Autodesk Fusion 360 part; units mm, degrees
(part 2 of 11)
  line L949 (170.706, 44.1166) -> (171.506, 44.1166)
  line L950 (171.506, 44.1166) -> (171.506, 43.1161)
  line L951 (171.506, 43.1161) -> (185.506, 43.1161)
  line L952 (185.506, 43.1161) -> (185.506, 44.1166)
  line L953 (185.506, 44.1166) -> (186.307, 44.1166)
  line L954 (186.307, 44.1166) -> (186.307, 47.2172)
  line L955 (186.307, 47.2172) -> (185.506, 47.2172)
  line L956 (185.506, 47.2172) -> (185.506, 53.0172)
  line L957 (185.506, 53.0172) -> (186.307, 53.0172)
  line L958 (186.307, 53.0172) -> (186.307, 56.1164)
  line L959 (186.307, 56.1164) -> (185.506, 56.1164)
  line L960 (185.506, 56.1164) -> (185.506, 57.1168)
  line L961 (185.506, 57.1168) -> (171.506, 57.1168)
  line L962 (190.556, 57.1168) -> (190.556, 56.1164)
  line L963 (190.556, 56.1164) -> (189.756, 56.1164)
  line L964 (189.756, 56.1164) -> (189.756, 53.0172)
  line L965 (189.756, 53.0172) -> (190.556, 53.0172)
  line L966 (190.556, 53.0172) -> (190.556, 47.2172)
  line L967 (190.556, 47.2172) -> (189.756, 47.2172)
  line L968 (189.756, 47.2172) -> (189.756, 44.1166)
  line L969 (189.756, 44.1166) -> (190.556, 44.1166)
  line L970 (190.556, 44.1166) -> (190.556, 43.1161)
  line L971 (190.556, 43.1161) -> (204.556, 43.1161)
  line L972 (204.556, 43.1161) -> (204.556, 44.1166)
  line L973 (204.556, 44.1166) -> (205.357, 44.1166)
  line L974 (205.357, 44.1166) -> (205.357, 47.2172)
  line L975 (205.357, 47.2172) -> (204.556, 47.2172)
  line L976 (204.556, 47.2172) -> (204.556, 53.0172)
  line L977 (204.556, 53.0172) -> (205.357, 53.0172)
  line L978 (205.357, 53.0172) -> (205.357, 56.1164)
  line L979 (205.357, 56.1164) -> (204.556, 56.1164)
  line L980 (204.556, 56.1164) -> (204.556, 57.1168)
  line L981 (204.556, 57.1168) -> (190.556, 57.1168)
  line L982 (209.606, 57.1168) -> (209.606, 56.1164)
  line L983 (209.606, 56.1164) -> (208.806, 56.1164)
  line L984 (208.806, 56.1164) -> (208.806, 53.0172)
  line L985 (208.806, 53.0172) -> (209.606, 53.0172)
  line L986 (209.606, 53.0172) -> (209.606, 47.2172)
  line L987 (209.606, 47.2172) -> (208.806, 47.2172)
  line L988 (208.806, 47.2172) -> (208.806, 44.1166)
  line L989 (208.806, 44.1166) -> (209.606, 44.1166)
  line L990 (209.606, 44.1166) -> (209.606, 43.1161)
  line L991 (209.606, 43.1161) -> (223.606, 43.1161)
  line L992 (223.606, 43.1161) -> (223.606, 44.1166)
  line L993 (223.606, 44.1166) -> (224.407, 44.1166)
  line L994 (224.407, 44.1166) -> (224.407, 47.2172)
  line L995 (224.407, 47.2172) -> (223.606, 47.2172)
  line L996 (223.606, 47.2172) -> (223.606, 53.0172)
  line L997 (223.606, 53.0172) -> (224.407, 53.0172)
  line L998 (224.407, 53.0172) -> (224.407, 56.1164)
  line L999 (224.407, 56.1164) -> (223.606, 56.1164)
  line L1000 (223.606, 56.1164) -> (223.606, 57.1168)
  line L1001 (223.606, 57.1168) -> (209.606, 57.1168)
  line L1002 (228.656, 57.1168) -> (228.656, 56.1164)
  line L1003 (228.656, 56.1164) -> (227.856, 56.1164)
  line L1004 (227.856, 56.1164) -> (227.856, 53.0172)
  line L1005 (227.856, 53.0172) -> (228.656, 53.0172)
  line L1006 (228.656, 53.0172) -> (228.656, 47.2172)
  line L1007 (228.656, 47.2172) -> (227.856, 47.2172)
  line L1008 (227.856, 47.2172) -> (227.856, 44.1166)
  line L1009 (227.856, 44.1166) -> (228.656, 44.1166)
  line L1010 (228.656, 44.1166) -> (228.656, 43.1161)
  line L1011 (228.656, 43.1161) -> (242.656, 43.1161)
  line L1012 (242.656, 43.1161) -> (242.656, 44.1166)
  line L1013 (242.656, 44.1166) -> (243.457, 44.1166)
  line L1014 (243.457, 44.1166) -> (243.457, 47.2172)
  line L1015 (243.457, 47.2172) -> (242.656, 47.2172)
  line L1016 (242.656, 47.2172) -> (242.656, 53.0172)
  line L1017 (242.656, 53.0172) -> (243.457, 53.0172)
  line L1018 (243.457, 53.0172) -> (243.457, 56.1164)
  line L1019 (243.457, 56.1164) -> (242.656, 56.1164)
  line L1020 (242.656, 56.1164) -> (242.656, 57.1168)
  line L1021 (242.656, 57.1168) -> (228.656, 57.1168)
  line L1022 (247.706, 57.1168) -> (247.706, 56.1164)
  line L1023 (247.706, 56.1164) -> (246.906, 56.1164)
  line L1024 (246.906, 56.1164) -> (246.906, 53.0172)
  line L1025 (246.906, 53.0172) -> (247.706, 53.0172)
  line L1026 (247.706, 53.0172) -> (247.706, 47.2172)
  line L1027 (247.706, 47.2172) -> (246.906, 47.2172)
  line L1028 (246.906, 47.2172) -> (246.906, 44.1166)
  line L1029 (246.906, 44.1166) -> (247.706, 44.1166)
  line L1030 (247.706, 44.1166) -> (247.706, 43.1161)
  line L1031 (247.706, 43.1161) -> (261.706, 43.1161)
  line L1032 (261.706, 43.1161) -> (261.706, 44.1166)
  line L1033 (261.706, 44.1166) -> (262.507, 44.1166)
  line L1034 (262.507, 44.1166) -> (262.507, 47.2172)
  line L1035 (262.507, 47.2172) -> (261.706, 47.2172)
  line L1036 (261.706, 47.2172) -> (261.706, 53.0172)
  line L1037 (261.706, 53.0172) -> (262.507, 53.0172)
  line L1038 (262.507, 53.0172) -> (262.507, 56.1164)
  line L1039 (262.507, 56.1164) -> (261.706, 56.1164)
  line L1040 (261.706, 56.1164) -> (261.706, 57.1168)
  line L1041 (261.706, 57.1168) -> (247.706, 57.1168)
  line L1042 (357.244, 57.1168) -> (357.244, 56.1164)
  line L1043 (357.244, 56.1164) -> (356.443, 56.1164)
  line L1044 (356.443, 56.1164) -> (356.443, 53.0172)
  line L1045 (356.443, 53.0172) -> (357.244, 53.0172)
  line L1046 (357.244, 53.0172) -> (357.244, 47.2172)
  line L1047 (357.244, 47.2172) -> (356.443, 47.2172)
  line L1048 (356.443, 47.2172) -> (356.443, 44.1166)
  line L1049 (356.443, 44.1166) -> (357.244, 44.1166)
  line L1050 (357.244, 44.1166) -> (357.244, 43.1161)
  line L1051 (357.244, 43.1161) -> (371.246, 43.1161)
  line L1052 (371.246, 43.1161) -> (371.246, 44.1166)
  line L1053 (371.246, 44.1166) -> (372.043, 44.1166)
  line L1054 (372.043, 44.1166) -> (372.043, 47.2172)
  line L1055 (372.043, 47.2172) -> (371.246, 47.2172)
  line L1056 (371.246, 47.2172) -> (371.246, 53.0172)
  line L1057 (371.246, 53.0172) -> (372.043, 53.0172)
  line L1058 (372.043, 53.0172) -> (372.043, 56.1164)
  line L1059 (372.043, 56.1164) -> (371.246, 56.1164)
  line L1060 (371.246, 56.1164) -> (371.246, 57.1168)
  line L1061 (371.246, 57.1168) -> (357.244, 57.1168)
  line L1062 (376.294, 57.1168) -> (376.294, 56.1164)
  line L1063 (376.294, 56.1164) -> (375.493, 56.1164)
  line L1064 (375.493, 56.1164) -> (375.493, 53.0172)
  line L1065 (375.493, 53.0172) -> (376.294, 53.0172)
  line L1066 (376.294, 53.0172) -> (376.294, 47.2172)
  line L1067 (376.294, 47.2172) -> (375.493, 47.2172)
  line L1068 (375.493, 47.2172) -> (375.493, 44.1166)
  line L1069 (375.493, 44.1166) -> (376.294, 44.1166)
  line L1070 (376.294, 44.1166) -> (376.294, 43.1161)
  line L1071 (376.294, 43.1161) -> (390.296, 43.1161)
  line L1072 (390.296, 43.1161) -> (390.296, 44.1166)
  line L1073 (390.296, 44.1166) -> (391.093, 44.1166)
  line L1074 (391.093, 44.1166) -> (391.093, 47.2172)
  line L1075 (391.093, 47.2172) -> (390.296, 47.2172)
  line L1076 (390.296, 47.2172) -> (390.296, 53.0172)
  line L1077 (390.296, 53.0172) -> (391.093, 53.0172)
  line L1078 (391.093, 53.0172) -> (391.093, 56.1164)
  line L1079 (391.093, 56.1164) -> (390.296, 56.1164)
  line L1080 (390.296, 56.1164) -> (390.296, 57.1168)
  line L1081 (390.296, 57.1168) -> (376.294, 57.1168)
  line L1082 (395.344, 57.1168) -> (395.344, 56.1164)
  line L1083 (395.344, 56.1164) -> (394.543, 56.1164)
  line L1084 (394.543, 56.1164) -> (394.543, 53.0172)
  line L1085 (394.543, 53.0172) -> (395.344, 53.0172)
  line L1086 (395.344, 53.0172) -> (395.344, 47.2172)
  line L1087 (395.344, 47.2172) -> (394.543, 47.2172)
  line L1088 (394.543, 47.2172) -> (394.543, 44.1166)
  line L1089 (394.543, 44.1166) -> (395.344, 44.1166)
  line L1090 (395.344, 44.1166) -> (395.344, 43.1161)
  line L1091 (395.344, 43.1161) -> (409.346, 43.1161)
  line L1092 (409.346, 43.1161) -> (409.346, 44.1166)
  line L1093 (409.346, 44.1166) -> (410.143, 44.1166)
  line L1094 (410.143, 44.1166) -> (410.143, 47.2172)
  line L1095 (410.143, 47.2172) -> (409.346, 47.2172)
  line L1096 (409.346, 47.2172) -> (409.346, 53.0172)
  line L1097 (409.346, 53.0172) -> (410.143, 53.0172)
  line L1098 (410.143, 53.0172) -> (410.143, 56.1164)
  line L1099 (410.143, 56.1164) -> (409.346, 56.1164)
  line L1100 (409.346, 56.1164) -> (409.346, 57.1168)
  line L1101 (409.346, 57.1168) -> (395.344, 57.1168)
  line L1102 (275.638, 75.741) -> (275.638, 74.9169)
  line L1103 (275.638, 74.9169) -> (269.368, 74.9169)
  line L1104 (269.368, 74.9169) -> (269.368, 73.1919)
  line L1105 (269.368, 73.1919) -> (268.388, 73.1919)
  line L1106 (268.388, 73.1919) -> (268.388, 69.8913)
  line L1107 (268.388, 69.8913) -> (269.368, 69.8913)
  line L1108 (269.368, 69.8913) -> (269.368, 68.1662)
  line L1109 (269.368, 68.1662) -> (273.837, 68.1662)
  line L1110 (273.837, 68.1662) -> (273.837, 66.6418)
  line L1111 (273.837, 66.6418) -> (273.237, 66.6418)
  line L1112 (273.237, 66.6418) -> (273.237, 67.4412)
  line L1113 (273.237, 67.4412) -> (270.137, 67.4412)
  line L1114 (270.137, 67.4412) -> (270.137, 66.6418)
  line L1115 (270.137, 66.6418) -> (269.138, 66.6418)
  line L1116 (269.138, 66.6418) -> (269.138, 52.6411)
  line L1117 (269.138, 52.6411) -> (270.137, 52.6411)
  line L1118 (270.137, 52.6411) -> (270.137, 51.8418)
  line L1119 (270.137, 51.8418) -> (273.237, 51.8418)
  line L1120 (273.237, 51.8418) -> (273.237, 52.6411)
  line L1121 (273.237, 52.6411) -> (273.837, 52.6411)
  line L1122 (273.837, 52.6411) -> (273.837, 51.1168)
  line L1123 (273.837, 51.1168) -> (269.368, 51.1168)
  line L1124 (269.368, 51.1168) -> (269.368, 49.3917)
  line L1125 (269.368, 49.3917) -> (268.388, 49.3917)
  line L1126 (268.388, 49.3917) -> (268.388, 46.0911)
  line L1127 (268.388, 46.0911) -> (269.368, 46.0911)
  line L1128 (269.368, 46.0911) -> (269.368, 44.366)
  line L1129 (269.368, 44.366) -> (275.638, 44.366)
  line L1130 (275.638, 44.366) -> (275.638, 43.542)
  line L1131 (275.638, 43.542) -> (278.438, 43.542)
  line L1132 (278.438, 43.542) -> (278.438, 44.366)
  line L1133 (278.438, 44.366) -> (281.667, 44.366)
  line L1134 (281.667, 44.366) -> (281.667, 46.0911)
  line L1135 (281.667, 46.0911) -> (282.587, 46.0911)
  line L1136 (282.587, 46.0911) -> (282.587, 49.3917)
  line L1137 (282.587, 49.3917) -> (281.667, 49.3917)
  line L1138 (281.667, 49.3917) -> (281.667, 51.1168)
  line L1139 (281.667, 51.1168) -> (278.438, 51.1168)
  line L1140 (278.438, 51.1168) -> (278.438, 52.6411)
  line L1141 (278.438, 52.6411) -> (279.038, 52.6411)
  line L1142 (279.038, 52.6411) -> (279.038, 51.8418)
  line L1143 (279.038, 51.8418) -> (282.138, 51.8418)
  line L1144 (282.138, 51.8418) -> (282.138, 52.6411)
  line L1145 (282.138, 52.6411) -> (283.137, 52.6411)
  line L1146 (283.137, 52.6411) -> (283.137, 66.6418)
  line L1147 (283.137, 66.6418) -> (282.138, 66.6418)
  line L1148 (282.138, 66.6418) -> (282.138, 67.4412)
  line L1149 (282.138, 67.4412) -> (279.038, 67.4412)
  line L1150 (279.038, 67.4412) -> (279.038, 66.6418)
  line L1151 (279.038, 66.6418) -> (278.438, 66.6418)
  line L1152 (278.438, 66.6418) -> (278.438, 68.1662)
  line L1153 (278.438, 68.1662) -> (281.667, 68.1662)
  line L1154 (281.667, 68.1662) -> (281.667, 69.8913)
  line L1155 (281.667, 69.8913) -> (282.587, 69.8913)
  line L1156 (282.587, 69.8913) -> (282.587, 73.1919)
  line L1157 (282.587, 73.1919) -> (281.667, 73.1919)
  line L1158 (281.667, 73.1919) -> (281.667, 74.9169)
  line L1159 (281.667, 74.9169) -> (278.438, 74.9169)
  line L1160 (278.438, 74.9169) -> (278.438, 75.741)
  line L1161 (278.438, 75.741) -> (275.638, 75.741)
  line L1162 (420.896, 75.741) -> (420.896, 74.9169)
  line L1163 (420.896, 74.9169) -> (414.623, 74.9169)
  line L1164 (414.623, 74.9169) -> (414.623, 73.1919)
  line L1165 (414.623, 73.1919) -> (413.646, 73.1919)
  line L1166 (413.646, 73.1919) -> (413.646, 69.8913)
  line L1167 (413.646, 69.8913) -> (414.623, 69.8913)
  line L1168 (414.623, 69.8913) -> (414.623, 68.1662)
  line L1169 (414.623, 68.1662) -> (419.093, 68.1662)
  line L1170 (419.093, 68.1662) -> (419.093, 66.6418)
  line L1171 (419.093, 66.6418) -> (418.497, 66.6418)
  line L1172 (418.497, 66.6418) -> (418.497, 67.4412)
  line L1173 (418.497, 67.4412) -> (415.396, 67.4412)
  line L1174 (415.396, 67.4412) -> (415.396, 66.6418)
  line L1175 (415.396, 66.6418) -> (414.394, 66.6418)
  line L1176 (414.394, 66.6418) -> (414.394, 52.6411)
  line L1177 (414.394, 52.6411) -> (415.396, 52.6411)
  line L1178 (415.396, 52.6411) -> (415.396, 51.8418)
  line L1179 (415.396, 51.8418) -> (418.497, 51.8418)
  line L1180 (418.497, 51.8418) -> (418.497, 52.6411)
  line L1181 (418.497, 52.6411) -> (419.093, 52.6411)
  line L1182 (419.093, 52.6411) -> (419.093, 51.1168)
  line L1183 (419.093, 51.1168) -> (414.623, 51.1168)
  line L1184 (414.623, 51.1168) -> (414.623, 49.3917)
  line L1185 (414.623, 49.3917) -> (413.646, 49.3917)
  line L1186 (413.646, 49.3917) -> (413.646, 46.0911)
  line L1187 (413.646, 46.0911) -> (414.623, 46.0911)
  line L1188 (414.623, 46.0911) -> (414.623, 44.366)
  line L1189 (414.623, 44.366) -> (420.896, 44.366)
  line L1190 (420.896, 44.366) -> (420.896, 43.542)
  line L1191 (420.896, 43.542) -> (423.693, 43.542)
  line L1192 (423.693, 43.542) -> (423.693, 44.366)
  line L1193 (423.693, 44.366) -> (426.925, 44.366)
  line L1194 (426.925, 44.366) -> (426.925, 46.0911)
  line L1195 (426.925, 46.0911) -> (427.845, 46.0911)
  line L1196 (427.845, 46.0911) -> (427.845, 49.3917)
  line L1197 (427.845, 49.3917) -> (426.925, 49.3917)
  line L1198 (426.925, 49.3917) -> (426.925, 51.1168)
  line L1199 (426.925, 51.1168) -> (423.693, 51.1168)
  line L1200 (423.693, 51.1168) -> (423.693, 52.6411)
  line L1201 (423.693, 52.6411) -> (424.293, 52.6411)
  line L1202 (424.293, 52.6411) -> (424.293, 51.8418)
  line L1203 (424.293, 51.8418) -> (427.394, 51.8418)
  line L1204 (427.394, 51.8418) -> (427.394, 52.6411)
  line L1205 (427.394, 52.6411) -> (428.396, 52.6411)
  line L1206 (428.396, 52.6411) -> (428.396, 66.6418)
  line L1207 (428.396, 66.6418) -> (427.394, 66.6418)
  line L1208 (427.394, 66.6418) -> (427.394, 67.4412)
  line L1209 (427.394, 67.4412) -> (424.293, 67.4412)
  line L1210 (424.293, 67.4412) -> (424.293, 66.6418)
  line L1211 (424.293, 66.6418) -> (423.693, 66.6418)
  line L1212 (423.693, 66.6418) -> (423.693, 68.1662)
  line L1213 (423.693, 68.1662) -> (426.925, 68.1662)
  line L1214 (426.925, 68.1662) -> (426.925, 69.8913)
  line L1215 (426.925, 69.8913) -> (427.845, 69.8913)
  line L1216 (427.845, 69.8913) -> (427.845, 73.1919)
  line L1217 (427.845, 73.1919) -> (426.925, 73.1919)
  line L1218 (426.925, 73.1919) -> (426.925, 74.9169)
  line L1219 (426.925, 74.9169) -> (423.693, 74.9169)
  line L1220 (423.693, 74.9169) -> (423.693, 75.741)
  line L1221 (423.693, 75.741) -> (420.896, 75.741)
  line L1222 (9.5815, 76.1668) -> (9.5815, 75.1664)
  line L1223 (9.5815, 75.1664) -> (8.7808, 75.1664)
  line L1224 (8.7809, 75.1664) -> (8.7809, 72.0672)
  line L1225 (8.7809, 72.0672) -> (9.5815, 72.0672)
  line L1226 (9.5815, 72.0672) -> (9.5815, 66.2672)
  line L1227 (9.5815, 66.2672) -> (8.7808, 66.2672)
  line L1228 (8.7809, 66.2672) -> (8.7809, 63.1666)
  line L1229 (8.7809, 63.1666) -> (9.5815, 63.1666)
  line L1230 (9.5815, 63.1666) -> (9.5815, 62.1661)
  line L1231 (9.5815, 62.1661) -> (23.581, 62.1661)
  line L1232 (23.581, 62.1661) -> (23.581, 63.1666)
  line L1233 (23.581, 63.1666) -> (24.3816, 63.1666)
  line L1234 (24.3816, 63.1666) -> (24.3816, 66.2672)
  line L1235 (24.3816, 66.2672) -> (23.581, 66.2672)
  line L1236 (23.581, 66.2672) -> (23.581, 72.0672)
  line L1237 (23.581, 72.0672) -> (24.3816, 72.0672)
  line L1238 (24.3816, 72.0672) -> (24.3816, 75.1664)
  line L1239 (24.3816, 75.1664) -> (23.581, 75.1664)
  line L1240 (23.581, 75.1664) -> (23.581, 76.1668)
  line L1241 (23.581, 76.1668) -> (9.5815, 76.1668)
  line L1242 (33.394, 76.1668) -> (33.394, 75.1664)
  line L1243 (33.394, 75.1664) -> (32.5947, 75.1664)
  line L1244 (32.5947, 75.1664) -> (32.5947, 72.0672)
  line L1245 (32.5947, 72.0672) -> (33.394, 72.0672)
  line L1246 (33.394, 72.0672) -> (33.394, 66.2672)
  line L1247 (33.394, 66.2672) -> (32.5947, 66.2672)
  line L1248 (32.5947, 66.2672) -> (32.5947, 63.1666)
  line L1249 (32.5947, 63.1666) -> (33.394, 63.1666)
  line L1250 (33.394, 63.1666) -> (33.394, 62.1661)
  line L1251 (33.394, 62.1661) -> (47.395, 62.1661)
  line L1252 (47.395, 62.1661) -> (47.395, 63.1666)
  line L1253 (47.395, 63.1666) -> (48.194, 63.1666)
  line L1254 (48.194, 63.1666) -> (48.194, 66.2672)
  line L1255 (48.194, 66.2672) -> (47.395, 66.2672)
  line L1256 (47.395, 66.2672) -> (47.395, 72.0672)
  line L1257 (47.395, 72.0672) -> (48.194, 72.0672)
  line L1258 (48.194, 72.0672) -> (48.194, 75.1664)
  line L1259 (48.194, 75.1664) -> (47.395, 75.1664)
  line L1260 (47.395, 75.1664) -> (47.395, 76.1668)
  line L1261 (47.395, 76.1668) -> (33.394, 76.1668)
  line L1262 (52.4439, 76.1668) -> (52.4439, 75.1664)
  line L1263 (52.4439, 75.1664) -> (51.6449, 75.1664)
  line L1264 (51.6449, 75.1664) -> (51.6449, 72.0672)
  line L1265 (51.6449, 72.0672) -> (52.4439, 72.0672)
  line L1266 (52.4439, 72.0672) -> (52.4439, 66.2672)
  line L1267 (52.4439, 66.2672) -> (51.6449, 66.2672)
  line L1268 (51.6449, 66.2672) -> (51.6449, 63.1666)
  line L1269 (51.6449, 63.1666) -> (52.4439, 63.1666)
  line L1270 (52.4439, 63.1666) -> (52.4439, 62.1661)
  line L1271 (52.4439, 62.1661) -> (66.445, 62.1661)
  line L1272 (66.445, 62.1661) -> (66.445, 63.1666)
  line L1273 (66.445, 63.1666) -> (67.244, 63.1666)
  line L1274 (67.244, 63.1666) -> (67.244, 66.2672)
  line L1275 (67.244, 66.2672) -> (66.445, 66.2672)
  line L1276 (66.445, 66.2672) -> (66.445, 72.0672)
  line L1277 (66.445, 72.0672) -> (67.244, 72.0672)
  line L1278 (67.244, 72.0672) -> (67.244, 75.1664)
  line L1279 (67.244, 75.1664) -> (66.445, 75.1664)
  line L1280 (66.445, 75.1664) -> (66.445, 76.1668)
  line L1281 (66.445, 76.1668) -> (52.4439, 76.1668)
  line L1282 (71.4939, 76.1668) -> (71.4939, 75.1664)
  line L1283 (71.4939, 75.1664) -> (70.6949, 75.1664)
  line L1284 (70.6949, 75.1664) -> (70.6949, 72.0672)
  line L1285 (70.6949, 72.0672) -> (71.4939, 72.0672)
  line L1286 (71.4939, 72.0672) -> (71.4939, 66.2672)
  line L1287 (71.4939, 66.2672) -> (70.6949, 66.2672)
  line L1288 (70.6949, 66.2672) -> (70.6949, 63.1666)
  line L1289 (70.6949, 63.1666) -> (71.4939, 63.1666)
  line L1290 (71.4939, 63.1666) -> (71.4939, 62.1661)
  line L1291 (71.4939, 62.1661) -> (85.4936, 62.1661)
  line L1292 (85.4936, 62.1661) -> (85.4936, 63.1666)
  line L1293 (85.4936, 63.1666) -> (86.294, 63.1666)
  line L1294 (86.294, 63.1666) -> (86.294, 66.2672)
  line L1295 (86.294, 66.2672) -> (85.4936, 66.2672)
  line L1296 (85.4936, 66.2672) -> (85.4936, 72.0672)
  line L1297 (85.4936, 72.0672) -> (86.294, 72.0672)
  line L1298 (86.294, 72.0672) -> (86.294, 75.1664)
  line L1299 (86.294, 75.1664) -> (85.4936, 75.1664)
  line L1300 (85.4936, 75.1664) -> (85.4936, 76.1668)
  line L1301 (85.4936, 76.1668) -> (71.4939, 76.1668)
  line L1302 (90.5439, 76.1668) -> (90.5439, 75.1664)
  line L1303 (90.5439, 75.1664) -> (89.7435, 75.1664)
  line L1304 (89.7435, 75.1664) -> (89.7435, 72.0672)
  line L1305 (89.7435, 72.0672) -> (90.5439, 72.0672)
  line L1306 (90.5439, 72.0672) -> (90.5439, 66.2672)
  line L1307 (90.5439, 66.2672) -> (89.7435, 66.2672)
  line L1308 (89.7435, 66.2672) -> (89.7435, 63.1666)
  line L1309 (89.7435, 63.1666) -> (90.5439, 63.1666)
  line L1310 (90.5439, 63.1666) -> (90.5439, 62.1661)
  line L1311 (90.5439, 62.1661) -> (104.544, 62.1661)
  line L1312 (104.544, 62.1661) -> (104.544, 63.1666)
  line L1313 (104.544, 63.1666) -> (105.344, 63.1666)
  line L1314 (105.344, 63.1666) -> (105.344, 66.2672)
  line L1315 (105.344, 66.2672) -> (104.544, 66.2672)
  line L1316 (104.544, 66.2672) -> (104.544, 72.0672)
  line L1317 (104.544, 72.0672) -> (105.344, 72.0672)
  line L1318 (105.344, 72.0672) -> (105.344, 75.1664)
  line L1319 (105.344, 75.1664) -> (104.544, 75.1664)
  line L1320 (104.544, 75.1664) -> (104.544, 76.1668)
  line L1321 (104.544, 76.1668) -> (90.5439, 76.1668)
  line L1322 (109.594, 76.1668) -> (109.594, 75.1664)
  line L1323 (109.594, 75.1664) -> (108.793, 75.1664)
  line L1324 (108.793, 75.1664) -> (108.793, 72.0672)
  line L1325 (108.793, 72.0672) -> (109.594, 72.0672)
  line L1326 (109.594, 72.0672) -> (109.594, 66.2672)
  line L1327 (109.594, 66.2672) -> (108.793, 66.2672)
  line L1328 (108.793, 66.2672) -> (108.793, 63.1666)
  line L1329 (108.793, 63.1666) -> (109.594, 63.1666)
  line L1330 (109.594, 63.1666) -> (109.594, 62.1661)
  line L1331 (109.594, 62.1661) -> (123.595, 62.1661)
  line L1332 (123.595, 62.1661) -> (123.595, 63.1666)
  line L1333 (123.595, 63.1666) -> (124.394, 63.1666)
  line L1334 (124.394, 63.1666) -> (124.394, 66.2672)
  line L1335 (124.394, 66.2672) -> (123.595, 66.2672)
  line L1336 (123.595, 66.2672) -> (123.595, 72.0672)
  line L1337 (123.595, 72.0672) -> (124.394, 72.0672)
  line L1338 (124.394, 72.0672) -> (124.394, 75.1664)
  line L1339 (124.394, 75.1664) -> (123.595, 75.1664)
  line L1340 (123.595, 75.1664) -> (123.595, 76.1668)
  line L1341 (123.595, 76.1668) -> (109.594, 76.1668)
  line L1342 (128.644, 76.1668) -> (128.644, 75.1664)
  line L1343 (128.644, 75.1664) -> (127.843, 75.1664)
  line L1344 (127.843, 75.1664) -> (127.843, 72.0672)
  line L1345 (127.843, 72.0672) -> (128.644, 72.0672)
  line L1346 (128.644, 72.0672) -> (128.644, 66.2672)
  line L1347 (128.644, 66.2672) -> (127.843, 66.2672)
  line L1348 (127.843, 66.2672) -> (127.843, 63.1666)
  line L1349 (127.843, 63.1666) -> (128.644, 63.1666)
  line L1350 (128.644, 63.1666) -> (128.644, 62.1661)
  line L1351 (128.644, 62.1661) -> (142.644, 62.1661)
  line L1352 (142.644, 62.1661) -> (142.644, 63.1666)
  line L1353 (142.644, 63.1666) -> (143.444, 63.1666)
  line L1354 (143.444, 63.1666) -> (143.444, 66.2672)
  line L1355 (143.444, 66.2672) -> (142.644, 66.2672)
  line L1356 (142.644, 66.2672) -> (142.644, 72.0672)
  line L1357 (142.644, 72.0672) -> (143.444, 72.0672)
  line L1358 (143.444, 72.0672) -> (143.444, 75.1664)
  line L1359 (143.444, 75.1664) -> (142.644, 75.1664)
  line L1360 (142.644, 75.1664) -> (142.644, 76.1668)
  line L1361 (142.644, 76.1668) -> (128.644, 76.1668)
  line L1362 (147.694, 76.1668) -> (147.694, 75.1664)
  line L1363 (147.694, 75.1664) -> (146.893, 75.1664)
  line L1364 (146.893, 75.1664) -> (146.893, 72.0672)
  line L1365 (146.893, 72.0672) -> (147.694, 72.0672)
  line L1366 (147.694, 72.0672) -> (147.694, 66.2672)
  line L1367 (147.694, 66.2672) -> (146.893, 66.2672)
  line L1368 (146.893, 66.2672) -> (146.893, 63.1666)
  line L1369 (146.893, 63.1666) -> (147.694, 63.1666)
  line L1370 (147.694, 63.1666) -> (147.694, 62.1661)
  line L1371 (147.694, 62.1661) -> (161.695, 62.1661)
  line L1372 (161.695, 62.1661) -> (161.695, 63.1666)
  line L1373 (161.695, 63.1666) -> (162.494, 63.1666)
  line L1374 (162.494, 63.1666) -> (162.494, 66.2672)
  line L1375 (162.494, 66.2672) -> (161.695, 66.2672)
  line L1376 (161.695, 66.2672) -> (161.695, 72.0672)
  line L1377 (161.695, 72.0672) -> (162.494, 72.0672)
  line L1378 (162.494, 72.0672) -> (162.494, 75.1664)
  line L1379 (162.494, 75.1664) -> (161.695, 75.1664)
  line L1380 (161.695, 75.1664) -> (161.695, 76.1668)
  line L1381 (161.695, 76.1668) -> (147.694, 76.1668)
  line L1382 (166.744, 76.1668) -> (166.744, 75.1664)
  line L1383 (166.744, 75.1664) -> (165.945, 75.1664)
  line L1384 (165.945, 75.1664) -> (165.945, 72.0672)
  line L1385 (165.945, 72.0672) -> (166.744, 72.0672)
  line L1386 (166.744, 72.0672) -> (166.744, 66.2672)
  line L1387 (166.744, 66.2672) -> (165.945, 66.2672)
  line L1388 (165.945, 66.2672) -> (165.945, 63.1666)
  line L1389 (165.945, 63.1666) -> (166.744, 63.1666)
  line L1390 (166.744, 63.1666) -> (166.744, 62.1661)
  line L1391 (166.744, 62.1661) -> (180.745, 62.1661)
  line L1392 (180.745, 62.1661) -> (180.745, 63.1666)
  line L1393 (180.745, 63.1666) -> (181.544, 63.1666)
  line L1394 (181.544, 63.1666) -> (181.544, 66.2672)
  line L1395 (181.544, 66.2672) -> (180.745, 66.2672)
  line L1396 (180.745, 66.2672) -> (180.745, 72.0672)
  line L1397 (180.745, 72.0672) -> (181.544, 72.0672)
  line L1398 (181.544, 72.0672) -> (181.544, 75.1664)
  line L1399 (181.544, 75.1664) -> (180.745, 75.1664)
  line L1400 (180.745, 75.1664) -> (180.745, 76.1668)
  line L1401 (180.745, 76.1668) -> (166.744, 76.1668)
  line L1402 (185.794, 76.1668) -> (185.794, 75.1664)
  line L1403 (185.794, 75.1664) -> (184.995, 75.1664)
  line L1404 (184.995, 75.1664) -> (184.995, 72.0672)
  line L1405 (184.995, 72.0672) -> (185.794, 72.0672)
  line L1406 (185.794, 72.0672) -> (185.794, 66.2672)
  line L1407 (185.794, 66.2672) -> (184.995, 66.2672)
  line L1408 (184.995, 66.2672) -> (184.995, 63.1666)
  line L1409 (184.995, 63.1666) -> (185.794, 63.1666)
  line L1410 (185.794, 63.1666) -> (185.794, 62.1661)
  line L1411 (185.794, 62.1661) -> (199.795, 62.1661)
  line L1412 (199.795, 62.1661) -> (199.795, 63.1666)
  line L1413 (199.795, 63.1666) -> (200.594, 63.1666)
  line L1414 (200.594, 63.1666) -> (200.594, 66.2672)
  line L1415 (200.594, 66.2672) -> (199.795, 66.2672)
  line L1416 (199.795, 66.2672) -> (199.795, 72.0672)
  line L1417 (199.795, 72.0672) -> (200.594, 72.0672)
  line L1418 (200.594, 72.0672) -> (200.594, 75.1664)
  line L1419 (200.594, 75.1664) -> (199.795, 75.1664)
  line L1420 (199.795, 75.1664) -> (199.795, 76.1668)
  line L1421 (199.795, 76.1668) -> (185.794, 76.1668)
  line L1422 (204.844, 76.1668) -> (204.844, 75.1664)
  line L1423 (204.844, 75.1664) -> (204.045, 75.1664)
  line L1424 (204.045, 75.1664) -> (204.045, 72.0672)
  line L1425 (204.045, 72.0672) -> (204.844, 72.0672)
  line L1426 (204.844, 72.0672) -> (204.844, 66.2672)
  line L1427 (204.844, 66.2672) -> (204.045, 66.2672)
  line L1428 (204.045, 66.2672) -> (204.045, 63.1666)
  line L1429 (204.045, 63.1666) -> (204.844, 63.1666)
  line L1430 (204.844, 63.1666) -> (204.844, 62.1661)
  line L1431 (204.844, 62.1661) -> (218.845, 62.1661)
  line L1432 (218.845, 62.1661) -> (218.845, 63.1666)
  line L1433 (218.845, 63.1666) -> (219.644, 63.1666)
  line L1434 (219.644, 63.1666) -> (219.644, 66.2672)
  line L1435 (219.644, 66.2672) -> (218.845, 66.2672)
  line L1436 (218.845, 66.2672) -> (218.845, 72.0672)
  line L1437 (218.845, 72.0672) -> (219.644, 72.0672)
  line L1438 (219.644, 72.0672) -> (219.644, 75.1664)
  line L1439 (219.644, 75.1664) -> (218.845, 75.1664)
  line L1440 (218.845, 75.1664) -> (218.845, 76.1668)
  line L1441 (218.845, 76.1668) -> (204.844, 76.1668)
  line L1442 (223.894, 76.1668) -> (223.894, 75.1664)
  line L1443 (223.894, 75.1664) -> (223.095, 75.1664)
  line L1444 (223.095, 75.1664) -> (223.095, 72.0672)
  line L1445 (223.095, 72.0672) -> (223.894, 72.0672)
  line L1446 (223.894, 72.0672) -> (223.894, 66.2672)
  line L1447 (223.894, 66.2672) -> (223.095, 66.2672)
  line L1448 (223.095, 66.2672) -> (223.095, 63.1666)
  line L1449 (223.095, 63.1666) -> (223.894, 63.1666)
  line L1450 (223.894, 63.1666) -> (223.894, 62.1661)
  line L1451 (223.894, 62.1661) -> (237.895, 62.1661)
  line L1452 (237.895, 62.1661) -> (237.895, 63.1666)
  line L1453 (237.895, 63.1666) -> (238.694, 63.1666)
  line L1454 (238.694, 63.1666) -> (238.694, 66.2672)
  line L1455 (238.694, 66.2672) -> (237.895, 66.2672)
  line L1456 (237.895, 66.2672) -> (237.895, 72.0672)
  line L1457 (237.895, 72.0672) -> (238.694, 72.0672)
  line L1458 (238.694, 72.0672) -> (238.694, 75.1664)
  line L1459 (238.694, 75.1664) -> (237.895, 75.1664)
  line L1460 (237.895, 75.1664) -> (237.895, 76.1668)
  line L1461 (237.895, 76.1668) -> (223.894, 76.1668)
  line L1462 (242.944, 76.1668) -> (242.944, 75.1664)
  line L1463 (242.944, 75.1664) -> (242.145, 75.1664)
  line L1464 (242.145, 75.1664) -> (242.145, 72.0672)
  line L1465 (242.145, 72.0672) -> (242.944, 72.0672)
  line L1466 (242.944, 72.0672) -> (242.944, 66.2672)
  line L1467 (242.944, 66.2672) -> (242.145, 66.2672)
  line L1468 (242.145, 66.2672) -> (242.145, 63.1666)
  line L1469 (242.145, 63.1666) -> (242.944, 63.1666)
  line L1470 (242.944, 63.1666) -> (242.944, 62.1661)
  line L1471 (242.944, 62.1661) -> (256.945, 62.1661)
  line L1472 (256.945, 62.1661) -> (256.945, 63.1666)
  line L1473 (256.945, 63.1666) -> (257.744, 63.1666)
  line L1474 (257.744, 63.1666) -> (257.744, 66.2672)
  line L1475 (257.744, 66.2672) -> (256.945, 66.2672)
  line L1476 (256.945, 66.2672) -> (256.945, 72.0672)
  line L1477 (256.945, 72.0672) -> (257.744, 72.0672)
  line L1478 (257.744, 72.0672) -> (257.744, 75.1664)
  line L1479 (257.744, 75.1664) -> (256.945, 75.1664)
  line L1480 (256.945, 75.1664) -> (256.945, 76.1668)
  line L1481 (256.945, 76.1668) -> (242.944, 76.1668)
  line L1482 (295.331, 76.1668) -> (295.331, 75.1664)
  line L1483 (295.331, 75.1664) -> (294.531, 75.1664)
  line L1484 (294.531, 75.1664) -> (294.531, 72.0672)
  line L1485 (294.531, 72.0672) -> (295.331, 72.0672)
  line L1486 (295.331, 72.0672) -> (295.331, 66.2672)
  line L1487 (295.331, 66.2672) -> (294.531, 66.2672)
  line L1488 (294.531, 66.2672) -> (294.531, 63.1666)
  line L1489 (294.531, 63.1666) -> (295.331, 63.1666)
  line L1490 (295.331, 63.1666) -> (295.331, 62.1661)
  line L1491 (295.331, 62.1661) -> (309.331, 62.1661)
  line L1492 (309.331, 62.1661) -> (309.331, 63.1666)
  line L1493 (309.331, 63.1666) -> (310.132, 63.1666)
  line L1494 (310.132, 63.1666) -> (310.132, 66.2672)
  line L1495 (310.132, 66.2672) -> (309.331, 66.2672)
  line L1496 (309.331, 66.2672) -> (309.331, 72.0672)
  line L1497 (309.331, 72.0672) -> (310.132, 72.0672)
  line L1498 (310.132, 72.0672) -> (310.132, 75.1664)
  line L1499 (310.132, 75.1664) -> (309.331, 75.1664)
  line L1500 (309.331, 75.1664) -> (309.331, 76.1668)
  line L1501 (309.331, 76.1668) -> (295.331, 76.1668)
  line L1502 (314.381, 76.1668) -> (314.381, 75.1664)
  line L1503 (314.381, 75.1664) -> (313.581, 75.1664)
  line L1504 (313.581, 75.1664) -> (313.581, 72.0672)
  line L1505 (313.581, 72.0672) -> (314.381, 72.0672)
  line L1506 (314.381, 72.0672) -> (314.381, 66.2672)
  line L1507 (314.381, 66.2672) -> (313.581, 66.2672)
  line L1508 (313.581, 66.2672) -> (313.581, 63.1666)
  line L1509 (313.581, 63.1666) -> (314.381, 63.1666)
  line L1510 (314.381, 63.1666) -> (314.381, 62.1661)
  line L1511 (314.381, 62.1661) -> (328.381, 62.1661)
  line L1512 (328.381, 62.1661) -> (328.381, 63.1666)
  line L1513 (328.381, 63.1666) -> (329.182, 63.1666)
  line L1514 (329.182, 63.1666) -> (329.182, 66.2672)
  line L1515 (329.182, 66.2672) -> (328.381, 66.2672)
  line L1516 (328.381, 66.2672) -> (328.381, 72.0672)
  line L1517 (328.381, 72.0672) -> (329.182, 72.0672)
  line L1518 (329.182, 72.0672) -> (329.182, 75.1664)
  line L1519 (329.182, 75.1664) -> (328.381, 75.1664)
  line L1520 (328.381, 75.1664) -> (328.381, 76.1668)
  line L1521 (328.381, 76.1668) -> (314.381, 76.1668)
  line L1522 (333.431, 76.1668) -> (333.431, 75.1664)
  line L1523 (333.431, 75.1664) -> (332.631, 75.1664)
  line L1524 (332.631, 75.1664) -> (332.631, 72.0672)
  line L1525 (332.631, 72.0672) -> (333.431, 72.0672)
  line L1526 (333.431, 72.0672) -> (333.431, 66.2672)
  line L1527 (333.431, 66.2672) -> (332.631, 66.2672)
  line L1528 (332.631, 66.2672) -> (332.631, 63.1666)
  line L1529 (332.631, 63.1666) -> (333.431, 63.1666)
  line L1530 (333.431, 63.1666) -> (333.431, 62.1661)
  line L1531 (333.431, 62.1661) -> (347.431, 62.1661)
  line L1532 (347.431, 62.1661) -> (347.431, 63.1666)
  line L1533 (347.431, 63.1666) -> (348.232, 63.1666)
  line L1534 (348.232, 63.1666) -> (348.232, 66.2672)
  line L1535 (348.232, 66.2672) -> (347.431, 66.2672)
  line L1536 (347.431, 66.2672) -> (347.431, 72.0672)
  line L1537 (347.431, 72.0672) -> (348.232, 72.0672)
  line L1538 (348.232, 72.0672) -> (348.232, 75.1664)
  line L1539 (348.232, 75.1664) -> (347.431, 75.1664)
  line L1540 (347.431, 75.1664) -> (347.431, 76.1668)
  line L1541 (347.431, 76.1668) -> (333.431, 76.1668)
  line L1542 (357.244, 76.1668) -> (357.244, 75.1664)
  line L1543 (357.244, 75.1664) -> (356.443, 75.1664)
  line L1544 (356.443, 75.1664) -> (356.443, 72.0672)
  line L1545 (356.443, 72.0672) -> (357.244, 72.0672)
  line L1546 (357.244, 72.0672) -> (357.244, 66.2672)
  line L1547 (357.244, 66.2672) -> (356.443, 66.2672)
  line L1548 (356.443, 66.2672) -> (356.443, 63.1666)
  line L1549 (356.443, 63.1666) -> (357.244, 63.1666)
  line L1550 (357.244, 63.1666) -> (357.244, 62.1661)
  line L1551 (357.244, 62.1661) -> (371.246, 62.1661)
  line L1552 (371.246, 62.1661) -> (371.246, 63.1666)
  line L1553 (371.246, 63.1666) -> (372.043, 63.1666)
  line L1554 (372.043, 63.1666) -> (372.043, 66.2672)
  line L1555 (372.043, 66.2672) -> (371.246, 66.2672)
  line L1556 (371.246, 66.2672) -> (371.246, 72.0672)
  line L1557 (371.246, 72.0672) -> (372.043, 72.0672)
  line L1558 (372.043, 72.0672) -> (372.043, 75.1664)
  line L1559 (372.043, 75.1664) -> (371.246, 75.1664)
  line L1560 (371.246, 75.1664) -> (371.246, 76.1668)
  line L1561 (371.246, 76.1668) -> (357.244, 76.1668)
  line L1562 (376.294, 76.1668) -> (376.294, 75.1664)
  line L1563 (376.294, 75.1664) -> (375.493, 75.1664)
  line L1564 (375.493, 75.1664) -> (375.493, 72.0672)
  line L1565 (375.493, 72.0672) -> (376.294, 72.0672)
  line L1566 (376.294, 72.0672) -> (376.294, 66.2672)
  line L1567 (376.294, 66.2672) -> (375.493, 66.2672)
  line L1568 (375.493, 66.2672) -> (375.493, 63.1666)
  line L1569 (375.493, 63.1666) -> (376.294, 63.1666)
  line L1570 (376.294, 63.1666) -> (376.294, 62.1661)
  line L1571 (376.294, 62.1661) -> (390.296, 62.1661)
  line L1572 (390.296, 62.1661) -> (390.296, 63.1666)
  line L1573 (390.296, 63.1666) -> (391.093, 63.1666)
  line L1574 (391.093, 63.1666) -> (391.093, 66.2672)
  line L1575 (391.093, 66.2672) -> (390.296, 66.2672)
  line L1576 (390.296, 66.2672) -> (390.296, 72.0672)
  line L1577 (390.296, 72.0672) -> (391.093, 72.0672)
  line L1578 (391.093, 72.0672) -> (391.093, 75.1664)
  line L1579 (391.093, 75.1664) -> (390.296, 75.1664)
  line L1580 (390.296, 75.1664) -> (390.296, 76.1668)
  line L1581 (390.296, 76.1668) -> (376.294, 76.1668)
  line L1582 (395.344, 76.1668) -> (395.344, 75.1664)
  line L1583 (395.344, 75.1664) -> (394.543, 75.1664)
  line L1584 (394.543, 75.1664) -> (394.543, 72.0672)
  line L1585 (394.543, 72.0672) -> (395.344, 72.0672)
  line L1586 (395.344, 72.0672) -> (395.344, 66.2672)
  line L1587 (395.344, 66.2672) -> (394.543, 66.2672)
  line L1588 (394.543, 66.2672) -> (394.543, 63.1666)
  line L1589 (394.543, 63.1666) -> (395.344, 63.1666)
  line L1590 (395.344, 63.1666) -> (395.344, 62.1661)
  line L1591 (395.344, 62.1661) -> (409.346, 62.1661)
  line L1592 (409.346, 62.1661) -> (409.346, 63.1666)
  line L1593 (409.346, 63.1666) -> (410.143, 63.1666)
  line L1594 (410.143, 63.1666) -> (410.143, 66.2672)
  line L1595 (410.143, 66.2672) -> (409.346, 66.2672)
  line L1596 (409.346, 66.2672) -> (409.346, 72.0672)
  line L1597 (409.346, 72.0672) -> (410.143, 72.0672)
  line L1598 (410.143, 72.0672) -> (410.143, 75.1664)
  line L1599 (410.143, 75.1664) -> (409.346, 75.1664)
  line L1600 (409.346, 75.1664) -> (409.346, 76.1668)
  line L1601 (409.346, 76.1668) -> (395.344, 76.1668)
  line L1602 (261.994, 95.2168) -> (261.994, 94.2164)
  line L1603 (261.994, 94.2164) -> (261.195, 94.2164)
  line L1604 (261.195, 94.2164) -> (261.195, 91.1172)
  line L1605 (261.195, 91.1172) -> (261.994, 91.1172)
  line L1606 (261.994, 91.1172) -> (261.994, 90.5164)
  line L1607 (261.994, 90.5164) -> (260.47, 90.5164)
  line L1608 (260.47, 90.5164) -> (260.47, 93.7465)
  line L1609 (260.47, 93.7465) -> (258.745, 93.7465)
  line L1610 (258.745, 93.7465) -> (258.745, 94.6672)
  line L1611 (258.745, 94.6672) -> (255.444, 94.6672)
  line L1612 (255.444, 94.6672) -> (255.444, 93.7465)
  line L1613 (255.444, 93.7465) -> (253.719, 93.7465)
  line L1614 (253.719, 93.7465) -> (253.719, 90.5164)
  line L1615 (253.719, 90.5164) -> (252.895, 90.5164)
  line L1616 (252.895, 90.5164) -> (252.895, 87.7164)
  line L1617 (252.895, 87.7164) -> (253.719, 87.7164)
  line L1618 (253.719, 87.7164) -> (253.719, 81.4462)
  line L1619 (253.719, 81.4462) -> (255.444, 81.4462)
  line L1620 (255.444, 81.4462) -> (255.444, 80.4665)
  line L1621 (255.444, 80.4665) -> (258.745, 80.4665)
  line L1622 (258.745, 80.4665) -> (258.745, 81.4462)
  line L1623 (258.745, 81.4462) -> (260.47, 81.4462)
  line L1624 (260.47, 81.4462) -> (260.47, 85.9166)
  line L1625 (260.47, 85.9166) -> (261.994, 85.9166)
  line L1626 (261.994, 85.9166) -> (261.994, 85.3172)
  line L1627 (261.994, 85.3172) -> (261.195, 85.3172)
  line L1628 (261.195, 85.3172) -> (261.195, 82.2166)
  line L1629 (261.195, 82.2166) -> (261.994, 82.2166)
  line L1630 (261.994, 82.2166) -> (261.994, 81.2161)
  line L1631 (261.994, 81.2161) -> (275.995, 81.2161)
  line L1632 (275.995, 81.2161) -> (275.995, 82.2166)
  line L1633 (275.995, 82.2166) -> (276.794, 82.2166)
  line L1634 (276.794, 82.2166) -> (276.794, 85.3172)
  line L1635 (276.794, 85.3172) -> (275.995, 85.3172)
  line L1636 (275.995, 85.3172) -> (275.995, 85.9166)
  line L1637 (275.995, 85.9166) -> (277.519, 85.9166)
  line L1638 (277.519, 85.9166) -> (277.519, 81.4462)
  line L1639 (277.519, 81.4462) -> (279.244, 81.4462)
  line L1640 (279.244, 81.4462) -> (279.244, 80.4665)
  line L1641 (279.244, 80.4665) -> (282.545, 80.4665)
  line L1642 (282.545, 80.4665) -> (282.545, 81.4462)
  line L1643 (282.545, 81.4462) -> (284.27, 81.4462)
  line L1644 (284.27, 81.4462) -> (284.27, 87.7164)
  line L1645 (284.27, 87.7164) -> (285.094, 87.7164)
  line L1646 (285.094, 87.7164) -> (285.094, 90.5164)
  line L1647 (285.094, 90.5164) -> (284.27, 90.5164)
  line L1648 (284.27, 90.5164) -> (284.27, 93.7465)
  line L1649 (284.27, 93.7465) -> (282.545, 93.7465)
  line L1650 (282.545, 93.7465) -> (282.545, 94.6672)
  line L1651 (282.545, 94.6672) -> (279.244, 94.6672)
  line L1652 (279.244, 94.6672) -> (279.244, 93.7465)
  line L1653 (279.244, 93.7465) -> (277.519, 93.7465)
  line L1654 (277.519, 93.7465) -> (277.519, 90.5164)
  line L1655 (277.519, 90.5164) -> (275.995, 90.5164)
  line L1656 (275.995, 90.5164) -> (275.995, 91.1172)
  line L1657 (275.995, 91.1172) -> (276.794, 91.1172)
  line L1658 (276.794, 91.1172) -> (276.794, 94.2164)
  line L1659 (276.794, 94.2164) -> (275.995, 94.2164)
  line L1660 (275.995, 94.2164) -> (275.995, 95.2168)
  line L1661 (275.995, 95.2168) -> (261.994, 95.2168)
  line L1662 (4.819, 95.2168) -> (4.819, 94.2164)
  line L1663 (4.819, 94.2164) -> (4.0197, 94.2164)
  line L1664 (4.0197, 94.2164) -> (4.0197, 91.1172)
  line L1665 (4.0197, 91.1172) -> (4.819, 91.1172)
  line L1666 (4.819, 91.1172) -> (4.819, 85.3172)
  line L1667 (4.819, 85.3172) -> (4.0197, 85.3172)
  line L1668 (4.0197, 85.3172) -> (4.0197, 82.2166)
  line L1669 (4.0197, 82.2166) -> (4.819, 82.2166)
  line L1670 (4.819, 82.2166) -> (4.819, 81.2161)
  line L1671 (4.819, 81.2161) -> (18.8199, 81.2161)
  line L1672 (18.8199, 81.2161) -> (18.8199, 82.2166)
  line L1673 (18.8199, 82.2166) -> (19.6191, 82.2166)
  line L1674 (19.6191, 82.2166) -> (19.6191, 85.3172)
  line L1675 (19.6191, 85.3172) -> (18.8199, 85.3172)
  line L1676 (18.8199, 85.3172) -> (18.8199, 91.1172)
  line L1677 (18.8199, 91.1172) -> (19.6191, 91.1172)
  line L1678 (19.6191, 91.1172) -> (19.6191, 94.2164)
  line L1679 (19.6191, 94.2164) -> (18.8199, 94.2164)
  line L1680 (18.8199, 94.2164) -> (18.8199, 95.2168)
  line L1681 (18.8199, 95.2168) -> (4.819, 95.2168)
  line L1682 (23.869, 95.2168) -> (23.869, 94.2164)
  line L1683 (23.869, 94.2164) -> (23.0697, 94.2164)
  line L1684 (23.0697, 94.2164) -> (23.0697, 91.1172)
  line L1685 (23.0697, 91.1172) -> (23.869, 91.1172)
  line L1686 (23.869, 91.1172) -> (23.869, 85.3172)
  line L1687 (23.869, 85.3172) -> (23.0697, 85.3172)
  line L1688 (23.0697, 85.3172) -> (23.0697, 82.2166)
  line L1689 (23.0697, 82.2166) -> (23.869, 82.2166)
  line L1690 (23.869, 82.2166) -> (23.869, 81.2161)
  line L1691 (23.869, 81.2161) -> (37.87, 81.2161)
  line L1692 (37.87, 81.2161) -> (37.87, 82.2166)
  line L1693 (37.87, 82.2166) -> (38.669, 82.2166)
  line L1694 (38.669, 82.2166) -> (38.669, 85.3172)
  line L1695 (38.669, 85.3172) -> (37.87, 85.3172)
  line L1696 (37.87, 85.3172) -> (37.87, 91.1172)
  line L1697 (37.87, 91.1172) -> (38.669, 91.1172)
  line L1698 (38.669, 91.1172) -> (38.669, 94.2164)
  line L1699 (38.669, 94.2164) -> (37.87, 94.2164)
  line L1700 (37.87, 94.2164) -> (37.87, 95.2168)
  line L1701 (37.87, 95.2168) -> (23.869, 95.2168)
  line L1702 (42.9189, 95.2168) -> (42.9189, 94.2164)
  line L1703 (42.9189, 94.2164) -> (42.1199, 94.2164)
  line L1704 (42.1199, 94.2164) -> (42.1199, 91.1172)
  line L1705 (42.1199, 91.1172) -> (42.9189, 91.1172)
  line L1706 (42.9189, 91.1172) -> (42.9189, 85.3172)
  line L1707 (42.9189, 85.3172) -> (42.1199, 85.3172)
  line L1708 (42.1199, 85.3172) -> (42.1199, 82.2166)
  line L1709 (42.1199, 82.2166) -> (42.9189, 82.2166)
  line L1710 (42.9189, 82.2166) -> (42.9189, 81.2161)
  line L1711 (42.9189, 81.2161) -> (56.92, 81.2161)
  line L1712 (56.92, 81.2161) -> (56.92, 82.2166)
  line L1713 (56.92, 82.2166) -> (57.719, 82.2166)
  line L1714 (57.719, 82.2166) -> (57.719, 85.3172)
  line L1715 (57.719, 85.3172) -> (56.92, 85.3172)
  line L1716 (56.92, 85.3172) -> (56.92, 91.1172)
  line L1717 (56.92, 91.1172) -> (57.719, 91.1172)
  line L1718 (57.719, 91.1172) -> (57.719, 94.2164)
  line L1719 (57.719, 94.2164) -> (56.92, 94.2164)
  line L1720 (56.92, 94.2164) -> (56.92, 95.2168)
  line L1721 (56.92, 95.2168) -> (42.9189, 95.2168)
  line L1722 (61.9689, 95.2168) -> (61.9689, 94.2164)
  line L1723 (61.9689, 94.2164) -> (61.1699, 94.2164)
  line L1724 (61.1699, 94.2164) -> (61.1699, 91.1172)
  line L1725 (61.1699, 91.1172) -> (61.9689, 91.1172)
  line L1726 (61.9689, 91.1172) -> (61.9689, 85.3172)
  line L1727 (61.9689, 85.3172) -> (61.1699, 85.3172)
  line L1728 (61.1699, 85.3172) -> (61.1699, 82.2166)
  line L1729 (61.1699, 82.2166) -> (61.9689, 82.2166)
  line L1730 (61.9689, 82.2166) -> (61.9689, 81.2161)
  line L1731 (61.9689, 81.2161) -> (75.97, 81.2161)
  line L1732 (75.97, 81.2161) -> (75.97, 82.2166)
  line L1733 (75.97, 82.2166) -> (76.769, 82.2166)
  line L1734 (76.769, 82.2166) -> (76.769, 85.3172)
  line L1735 (76.769, 85.3172) -> (75.97, 85.3172)
  line L1736 (75.97, 85.3172) -> (75.97, 91.1172)
  line L1737 (75.97, 91.1172) -> (76.769, 91.1172)
  line L1738 (76.769, 91.1172) -> (76.769, 94.2164)
  line L1739 (76.769, 94.2164) -> (75.97, 94.2164)
  line L1740 (75.97, 94.2164) -> (75.97, 95.2168)
  line L1741 (75.97, 95.2168) -> (61.9689, 95.2168)
  line L1742 (81.0189, 95.2168) -> (81.0189, 94.2164)
  line L1743 (81.0189, 94.2164) -> (80.2199, 94.2164)
  line L1744 (80.2199, 94.2164) -> (80.2199, 91.1172)
  line L1745 (80.2199, 91.1172) -> (81.0189, 91.1172)
  line L1746 (81.0189, 91.1172) -> (81.0189, 85.3172)
  line L1747 (81.0189, 85.3172) -> (80.2199, 85.3172)
  line L1748 (80.2199, 85.3172) -> (80.2199, 82.2166)
  line L1749 (80.2199, 82.2166) -> (81.0189, 82.2166)
  line L1750 (81.0189, 82.2166) -> (81.0189, 81.2161)
  line L1751 (81.0189, 81.2161) -> (95.02, 81.2161)
  line L1752 (95.02, 81.2161) -> (95.02, 82.2166)
  line L1753 (95.02, 82.2166) -> (95.819, 82.2166)
  line L1754 (95.819, 82.2166) -> (95.819, 85.3172)
  line L1755 (95.819, 85.3172) -> (95.02, 85.3172)
  line L1756 (95.02, 85.3172) -> (95.02, 91.1172)
  line L1757 (95.02, 91.1172) -> (95.819, 91.1172)
  line L1758 (95.819, 91.1172) -> (95.819, 94.2164)
  line L1759 (95.819, 94.2164) -> (95.02, 94.2164)
  line L1760 (95.02, 94.2164) -> (95.02, 95.2168)
  line L1761 (95.02, 95.2168) -> (81.0189, 95.2168)
  line L1762 (100.069, 95.2168) -> (100.069, 94.2164)
  line L1763 (100.069, 94.2164) -> (99.2699, 94.2164)
  line L1764 (99.2699, 94.2164) -> (99.2699, 91.1172)
  line L1765 (99.2699, 91.1172) -> (100.069, 91.1172)
  line L1766 (100.069, 91.1172) -> (100.069, 85.3172)
  line L1767 (100.069, 85.3172) -> (99.2699, 85.3172)
  line L1768 (99.2699, 85.3172) -> (99.2699, 82.2166)
  line L1769 (99.2699, 82.2166) -> (100.069, 82.2166)
  line L1770 (100.069, 82.2166) -> (100.069, 81.2161)
  line L1771 (100.069, 81.2161) -> (114.07, 81.2161)
  line L1772 (114.07, 81.2161) -> (114.07, 82.2166)
  line L1773 (114.07, 82.2166) -> (114.869, 82.2166)
  line L1774 (114.869, 82.2166) -> (114.869, 85.3172)
  line L1775 (114.869, 85.3172) -> (114.07, 85.3172)
  line L1776 (114.07, 85.3172) -> (114.07, 91.1172)
  line L1777 (114.07, 91.1172) -> (114.869, 91.1172)
  line L1778 (114.869, 91.1172) -> (114.869, 94.2164)
  line L1779 (114.869, 94.2164) -> (114.07, 94.2164)
  line L1780 (114.07, 94.2164) -> (114.07, 95.2168)
  line L1781 (114.07, 95.2168) -> (100.069, 95.2168)
  line L1782 (119.119, 95.2168) -> (119.119, 94.2164)
  line L1783 (119.119, 94.2164) -> (118.32, 94.2164)
  line L1784 (118.32, 94.2164) -> (118.32, 91.1172)
  line L1785 (118.32, 91.1172) -> (119.119, 91.1172)
  line L1786 (119.119, 91.1172) -> (119.119, 85.3172)
  line L1787 (119.119, 85.3172) -> (118.32, 85.3172)
  line L1788 (118.32, 85.3172) -> (118.32, 82.2166)
  line L1789 (118.32, 82.2166) -> (119.119, 82.2166)
  line L1790 (119.119, 82.2166) -> (119.119, 81.2161)
  line L1791 (119.119, 81.2161) -> (133.12, 81.2161)
  line L1792 (133.12, 81.2161) -> (133.12, 82.2166)
  line L1793 (133.12, 82.2166) -> (133.919, 82.2166)
  line L1794 (133.919, 82.2166) -> (133.919, 85.3172)
  line L1795 (133.919, 85.3172) -> (133.12, 85.3172)
  line L1796 (133.12, 85.3172) -> (133.12, 91.1172)
  line L1797 (133.12, 91.1172) -> (133.919, 91.1172)
  line L1798 (133.919, 91.1172) -> (133.919, 94.2164)
  line L1799 (133.919, 94.2164) -> (133.12, 94.2164)
  line L1800 (133.12, 94.2164) -> (133.12, 95.2168)
  line L1801 (133.12, 95.2168) -> (119.119, 95.2168)
  line L1802 (138.169, 95.2168) -> (138.169, 94.2164)
  line L1803 (138.169, 94.2164) -> (137.37, 94.2164)
  line L1804 (137.37, 94.2164) -> (137.37, 91.1172)
  line L1805 (137.37, 91.1172) -> (138.169, 91.1172)
  line L1806 (138.169, 91.1172) -> (138.169, 85.3172)
  line L1807 (138.169, 85.3172) -> (137.37, 85.3172)
  line L1808 (137.37, 85.3172) -> (137.37, 82.2166)
  line L1809 (137.37, 82.2166) -> (138.169, 82.2166)
  line L1810 (138.169, 82.2166) -> (138.169, 81.2161)
  line L1811 (138.169, 81.2161) -> (152.17, 81.2161)
  line L1812 (152.17, 81.2161) -> (152.17, 82.2166)
  line L1813 (152.17, 82.2166) -> (152.969, 82.2166)
  line L1814 (152.969, 82.2166) -> (152.969, 85.3172)
  line L1815 (152.969, 85.3172) -> (152.17, 85.3172)
  line L1816 (152.17, 85.3172) -> (152.17, 91.1172)
  line L1817 (152.17, 91.1172) -> (152.969, 91.1172)
  line L1818 (152.969, 91.1172) -> (152.969, 94.2164)
  line L1819 (152.969, 94.2164) -> (152.17, 94.2164)
  line L1820 (152.17, 94.2164) -> (152.17, 95.2168)
  line L1821 (152.17, 95.2168) -> (138.169, 95.2168)
  line L1822 (157.219, 95.2168) -> (157.219, 94.2164)
  line L1823 (157.219, 94.2164) -> (156.42, 94.2164)
  line L1824 (156.42, 94.2164) -> (156.42, 91.1172)
  line L1825 (156.42, 91.1172) -> (157.219, 91.1172)
  line L1826 (157.219, 91.1172) -> (157.219, 85.3172)
  line L1827 (157.219, 85.3172) -> (156.42, 85.3172)
  line L1828 (156.42, 85.3172) -> (156.42, 82.2166)
  line L1829 (156.42, 82.2166) -> (157.219, 82.2166)
  line L1830 (157.219, 82.2166) -> (157.219, 81.2161)
  line L1831 (157.219, 81.2161) -> (171.22, 81.2161)
  line L1832 (171.22, 81.2161) -> (171.22, 82.2166)
  line L1833 (171.22, 82.2166) -> (172.019, 82.2166)
  line L1834 (172.019, 82.2166) -> (172.019, 85.3172)
  line L1835 (172.019, 85.3172) -> (171.22, 85.3172)
  line L1836 (171.22, 85.3172) -> (171.22, 91.1172)
  line L1837 (171.22, 91.1172) -> (172.019, 91.1172)
  line L1838 (172.019, 91.1172) -> (172.019, 94.2164)
  line L1839 (172.019, 94.2164) -> (171.22, 94.2164)
  line L1840 (171.22, 94.2164) -> (171.22, 95.2168)
  line L1841 (171.22, 95.2168) -> (157.219, 95.2168)
  line L1842 (176.269, 95.2168) -> (176.269, 94.2164)
  line L1843 (176.269, 94.2164) -> (175.47, 94.2164)
  line L1844 (175.47, 94.2164) -> (175.47, 91.1172)
  line L1845 (175.47, 91.1172) -> (176.269, 91.1172)
  line L1846 (176.269, 91.1172) -> (176.269, 85.3172)
  line L1847 (176.269, 85.3172) -> (175.47, 85.3172)
  line L1848 (175.47, 85.3172) -> (175.47, 82.2166)
  line L1849 (175.47, 82.2166) -> (176.269, 82.2166)
  line L1850 (176.269, 82.2166) -> (176.269, 81.2161)
  line L1851 (176.269, 81.2161) -> (190.27, 81.2161)
  line L1852 (190.27, 81.2161) -> (190.27, 82.2166)
  line L1853 (190.27, 82.2166) -> (191.069, 82.2166)
  line L1854 (191.069, 82.2166) -> (191.069, 85.3172)
  line L1855 (191.069, 85.3172) -> (190.27, 85.3172)
  line L1856 (190.27, 85.3172) -> (190.27, 91.1172)
  line L1857 (190.27, 91.1172) -> (191.069, 91.1172)
  line L1858 (191.069, 91.1172) -> (191.069, 94.2164)
  line L1859 (191.069, 94.2164) -> (190.27, 94.2164)
  line L1860 (190.27, 94.2164) -> (190.27, 95.2168)
  line L1861 (190.27, 95.2168) -> (176.269, 95.2168)
  line L1862 (195.319, 95.2168) -> (195.319, 94.2164)
  line L1863 (195.319, 94.2164) -> (194.52, 94.2164)
  line L1864 (194.52, 94.2164) -> (194.52, 91.1172)
  line L1865 (194.52, 91.1172) -> (195.319, 91.1172)
  line L1866 (195.319, 91.1172) -> (195.319, 85.3172)
  line L1867 (195.319, 85.3172) -> (194.52, 85.3172)
  line L1868 (194.52, 85.3172) -> (194.52, 82.2166)
  line L1869 (194.52, 82.2166) -> (195.319, 82.2166)
  line L1870 (195.319, 82.2166) -> (195.319, 81.2161)
  line L1871 (195.319, 81.2161) -> (209.32, 81.2161)
  line L1872 (209.32, 81.2161) -> (209.32, 82.2166)
  line L1873 (209.32, 82.2166) -> (210.119, 82.2166)
  line L1874 (210.119, 82.2166) -> (210.119, 85.3172)
  line L1875 (210.119, 85.3172) -> (209.32, 85.3172)
  line L1876 (209.32, 85.3172) -> (209.32, 91.1172)
  line L1877 (209.32, 91.1172) -> (210.119, 91.1172)
  line L1878 (210.119, 91.1172) -> (210.119, 94.2164)
  line L1879 (210.119, 94.2164) -> (209.32, 94.2164)
  line L1880 (209.32, 94.2164) -> (209.32, 95.2168)
  line L1881 (209.32, 95.2168) -> (195.319, 95.2168)